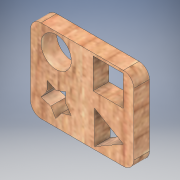
# Autodesk Inventor part: Passenger Base EM
Saved by Autodesk Inventor 2017 (Build 210142000, 142)
## iProperties
Created: 2020-02-14
Part Number: Passenger Base EM
Material: Wood (Birch)
Document SubType Name: Modeling
Designer: 10042265
Density: 0.55 g/cm^3
Appearance: Birch - Natural Polished
Author: 10042265
Autodesk Inventor part; units mm, degrees
ref_plane "YZ Plane" through (0, 0, 0) normal (1, 0, 0) x (0, 1, 0)
ref_plane "XZ Plane" through (0, 0, 0) normal (0, 1, 0) x (-1, 0, 0)
ref_plane "XY Plane" through (0, 0, 0) normal (0, 0, 1) x (1, 0, 0)
sketch "Sketch1" plane through (0, 0, 0) normal (0, 0, 1) x (1, 0, 0)
  line L0 (5.08, 0) -> (45.085, 0)
  line L1 (50.165, 5.08) -> (50.165, 35.306)
  line L2 (45.085, 40.386) -> (5.08, 40.386)
  line L3 (0, 35.306) -> (0, 5.08)
  arc A0 (5.08, 40.386) -> (0, 35.306) centre (5.08, 35.306) ccw
  arc A1 (0, 5.08) -> (5.08, 0) centre (5.08, 5.08) ccw
  arc A2 (45.085, 0) -> (50.165, 5.08) centre (45.085, 5.08) ccw
  arc A3 (50.165, 35.306) -> (45.085, 40.386) centre (45.085, 35.306) ccw
  point P0 (0, 0)
  point P1 (50.165, 0)
  point P2 (50.165, 40.386)
  dimension "d0" = 50.165
  dimension "d1" = 40.386
  dimension "d2" = 5.08
  constraints: 8 end point, 8 point on circle, 8 tangent, 6 point on line, 4 centre point, 3 equal radius, 2 perpendicular, 1 horizontal, 1 vertical
  measures "d0" distance of point (0, 0) point (50.165, 0)
  measures "d1" distance of point (50.165, 0) point (50.165, 40.386)
  measures "d2" radius of A0
extrude "Extrusion1" add sketch "Sketch1" along normal blind 7.62
sketch "Sketch2" plane through (0, 0, 7.62) normal (0, 0, 1) x (1, 0, 0)
  line L0 (0, 35.306) -> (0, 5.08) projected
  arc A0 (0, 5.08) -> (5.08, 0) centre (5.08, 5.08) ccw projected
  line L1 (5.08, 0) -> (45.085, 0) projected
  arc A1 (45.085, 0) -> (50.165, 5.08) centre (45.085, 5.08) ccw projected
  line L2 (50.165, 5.08) -> (50.165, 35.306) projected
  arc A2 (50.165, 35.306) -> (45.085, 40.386) centre (45.085, 35.306) ccw projected
  line L3 (45.085, 40.386) -> (5.08, 40.386) projected
  arc A3 (5.08, 40.386) -> (0, 35.306) centre (5.08, 35.306) ccw projected
  line L4 (45.085, 40.386) -> (5.08, 40.386) projected
  circle A4 centre (12.446, 31.75) radius 7.366
  line L5 (30.353, 39.116) -> (45.085, 39.116)
  line L6 (45.085, 39.116) -> (45.085, 24.384)
  line L7 (45.085, 24.384) -> (30.353, 24.384)
  line L8 (30.353, 24.384) -> (30.353, 39.116)
  line L9 (31.0509, 17.4752) -> (31.0509, 1.27)
  line L10 (31.0509, 1.27) -> (45.085, 9.3726)
  line L11 (45.085, 9.3726) -> (31.0509, 17.4752)
  circle A5 centre (12.446, 11.3013) radius 7.6835 construction
  line L12 (19.6887, 8.7364) -> (12.2447, 3.6204) construction
  line L13 (12.2447, 3.6204) -> (5.0789, 9.1192) construction
  line L14 (5.0789, 9.1192) -> (8.0941, 17.6336) construction
  line L15 (8.0941, 17.6336) -> (17.1235, 17.397) construction
  line L16 (17.1235, 17.397) -> (19.6887, 8.7364) construction
  line L17 (8.0941, 17.6336) -> (12.3737, 15.5731)
  line L18 (12.3737, 15.5731) -> (17.1235, 17.397)
  line L19 (17.1235, 17.397) -> (16.9991, 12.6499)
  line L20 (16.9991, 12.6499) -> (19.6887, 8.7364)
  line L21 (19.6887, 8.7364) -> (15.1335, 7.3908)
  line L22 (15.1335, 7.3908) -> (12.2447, 3.6204)
  line L23 (12.2447, 3.6204) -> (9.8287, 7.7099)
  line L24 (9.8287, 7.7099) -> (5.0789, 9.1192)
  line L25 (5.0789, 9.1192) -> (7.9752, 12.8838)
  line L26 (7.9752, 12.8838) -> (8.0941, 17.6336)
  point P0 (0, 0)
  dimension "d21" = 15.367
  dimension "d10" = 14.732
  dimension "d11" = 1.27
  dimension "d12" = 5.08
  dimension "d13" = 14.732
  dimension "d14" = 14.732
  dimension "d15" = 14.732
  dimension "d16" = 5.08
  dimension "d17" = 1.27
  dimension "d18" = 16.2052
  dimension "d19" = 5.08
  dimension "d20" = 1.27
  dimension "d23" = 4.7498
  dimension "d25" = 4.7498
  dimension "d26" = 4.7498
  dimension "d27" = 4.7498
  dimension "d28" = 4.7498
  dimension "d29" = 4.7498
  dimension "d30" = 4.7498
  dimension "d31" = 4.7498
  dimension "d32" = 4.747
  dimension "d33" = 3.9135
  constraints: 44 end point, 3 coincident, 2 equal length, 2 perpendicular, 1 centre point, 1 horizontal, 1 vertical, 14 other
  measures "d10" diameter of A4
  measures "d11" distance edge to line of A4 L3
  measures "d12" distance edge to line of A4 L0
  measures "d13" distance of L5.start L5.end
  measures "d14" distance of L5.end L6.end
  measures "d15" distance of L6.end L7.end
  measures "d16" distance between parallel lines of L2 L6
  measures "d17" distance between parallel lines of L3 L5
  measures "d18" distance of L9.start L9.end
  measures "d19" distance from line of L10.end L2
  measures "d20" distance from line of L9.end L1
  measures "d23" distance of L14.end L17.end
  measures "d25" distance of L12.start L21.end
  measures "d26" distance of L21.end L12.end
  measures "d27" distance of L12.end L23.end
  measures "d28" horizontal distance of L23.end L13.end
  measures "d29" vertical distance of L25.end L14.end
  measures "d30" distance of L13.end L25.end
  measures "d31" horizontal distance of L17.end L15.end
  measures "d32" vertical distance of L15.end L19.end
  measures "d33" vertical distance of L19.end L12.start
extrude "Extrusion2" cut sketch "Sketch2" against normal blind 7.62 contours A4 | L5 L6 L7 L8 | L11 L10 L9 | L17 L18 L19 L20 L21 L22 L23 L24 L25 L26
shell "Shell1" thickness 0.254 removed faces 1 at (40.407, 17.0773, 0)
body "Solid1"
